Autodesk Inventor part; units mm, degrees
(part 3 of 3)
sketch "Sketch7" plane through (4.7625, 0, 0) normal (1, 0, 0) x (0, 0, -1)
  arc A0 (177.1237, 146.6426) -> (185.0928, 143.4752) centre (181.8846, 147.0122) ccw projected
  line L0 (177.1237, 146.6426) -> (173.518, 193.0979) projected
  arc A1 (175.8624, 197.5861) -> (173.518, 193.0979) centre (178.2789, 193.4674) ccw projected
  arc A2 (175.8624, 197.5861) -> (177.263, 198.4856) centre (165.4189, 215.3861) ccw projected
  arc A3 (182.3196, 198.751) -> (177.263, 198.4856) centre (180.0035, 194.5751) ccw projected
  line L1 (182.3196, 198.751) -> (208.3567, 184.3098) projected
  arc A4 (210.3177, 182.2574) -> (208.3567, 184.3098) centre (206.0406, 180.1339) ccw projected
  arc A5 (210.3177, 182.2574) -> (211.6131, 180.3381) centre (218.1439, 186.1428) ccw projected
  arc A6 (212.7982, 177.6127) -> (211.6131, 180.3381) centre (208.044, 177.1657) ccw projected
  arc A7 (212.7982, 177.6127) -> (213.775, 174.2825) centre (221.8723, 178.4659) ccw projected
  arc A8 (212.7408, 168.5537) -> (213.775, 174.2825) centre (209.5326, 172.0906) ccw projected
  line L2 (212.7408, 168.5537) -> (185.0928, 143.4752) projected
  line L3 (297.693, 129.8322) -> (298.103, 129.6534) projected
  arc A9 (300.9106, 126.0225) -> (298.103, 129.6534) centre (296.1941, 125.2763) ccw projected
  arc A10 (300.9106, 126.0225) -> (303.4157, 119.6426) centre (316.6157, 128.5073) ccw projected
  arc A11 (303.9033, 115.2529) -> (303.4157, 119.6426) centre (299.4515, 116.9804) ccw projected
  arc A12 (301.9596, 113.1838) -> (303.9033, 115.2529) centre (299.6083, 117.34) ccw projected
  arc A13 (301.9596, 113.1838) -> (301.3812, 112.8276) centre (306.462, 105.2251) ccw projected
  arc A14 (298.4626, 112.03) -> (301.3812, 112.8276) centre (298.7279, 116.7978) ccw projected
  line L4 (298.4626, 112.03) -> (288.0097, 112.6116) projected
  arc A15 (284.8365, 120.693) -> (288.0097, 112.6116) centre (288.275, 117.3794) ccw projected
  line L5 (284.8365, 120.693) -> (292.1012, 128.2313) projected
  arc A16 (294.7827, 129.6326) -> (292.1012, 128.2313) centre (295.5396, 124.9178) ccw projected
  arc A17 (294.7827, 129.6326) -> (296.0335, 129.9248) centre (293.3334, 138.661) ccw projected
  arc A18 (297.693, 129.8322) -> (296.0335, 129.9248) centre (296.7386, 127.6436) ccw projected
  arc A19 (103.3374, 74.4504) -> (106.8132, 70.7682) centre (108.0195, 75.3885) ccw projected
  line L6 (103.3374, 74.4504) -> (95.1658, 115.2322) projected
  arc A20 (96.9547, 119.9692) -> (95.1658, 115.2322) centre (99.848, 116.1703) ccw projected
  arc A21 (96.9547, 119.9692) -> (101.5055, 124.7667) centre (84.4507, 136.3874) ccw projected
  arc A22 (106.1416, 126.803) -> (101.5055, 124.7667) centre (105.4517, 122.0779) ccw projected
  line L7 (106.1416, 126.803) -> (150.0332, 120.3943) projected
  arc A23 (152.7613, 112.3346) -> (150.0332, 120.3943) centre (149.3433, 115.6692) ccw projected
  line L8 (152.7613, 112.3346) -> (113.01, 71.5887) projected
  arc A24 (108.0902, 70.3904) -> (113.01, 71.5887) centre (109.5919, 74.9233) ccw projected
  arc A25 (108.0902, 70.3904) -> (106.8132, 70.7682) centre (101.6, 50.8) ccw projected
  arc A26 (79.5512, 19.1063) -> (80.7269, 11.5557) centre (82.9692, 15.7717) ccw projected
  line L9 (79.5512, 19.1063) -> (90.19, 30.0113) projected
  arc A27 (95.1098, 31.2096) -> (90.19, 30.0113) centre (93.6081, 26.6767) ccw projected
  arc A28 (95.1098, 31.2096) -> (99.5296, 30.2666) centre (101.6, 50.8) ccw projected
  arc A29 (103.5319, 27.1647) -> (99.5296, 30.2666) centre (99.0506, 25.5155) ccw projected
  line L10 (103.5319, 27.1647) -> (107.8479, 15.4373) projected
  arc A30 (107.879, 12.226) -> (107.8479, 15.4373) centre (103.3665, 13.7881) ccw projected
  arc A31 (107.879, 12.226) -> (107.4494, 10.4582) centre (116.952, 9.0853) ccw projected
  arc A32 (102.8585, 6.3678) -> (107.4494, 10.4582) centre (102.7233, 11.1411) ccw projected
  arc A33 (80.7269, 11.5557) -> (102.8585, 6.3678) centre (101.6, 50.8) ccw projected
  arc A34 (119.7664, 19.8236) -> (121.8244, 17.3583) centre (124.2477, 21.4729) ccw projected
  line L11 (119.7664, 19.8236) -> (115.4504, 31.551) projected
  arc A35 (116.4871, 36.5074) -> (115.4504, 31.551) centre (119.9318, 33.2003) ccw projected
  arc A36 (116.4871, 36.5074) -> (120.5052, 42.5235) centre (101.6, 50.8) ccw projected
  arc A37 (124.6863, 45.3797) -> (120.5052, 42.5235) centre (124.8796, 40.6084) ccw projected
  line L12 (124.6863, 45.3797) -> (179.7658, 47.6103) projected
  arc A38 (181.9351, 38.4919) -> (179.7658, 47.6103) centre (179.959, 42.839) ccw projected
  line L13 (181.9351, 38.4919) -> (129.3853, 14.6036) projected
  arc A39 (123.9358, 15.6738) -> (129.3853, 14.6036) centre (127.4092, 18.9507) ccw projected
  arc A40 (123.9358, 15.6738) -> (121.8244, 17.3583) centre (116.952, 9.0853) ccw projected
  arc A41 (269.7893, 127.2498) -> (264.2711, 128.2398) centre (263.4194, 107.6199) ccw projected
  arc A42 (260.0922, 131.0994) -> (264.2711, 128.2398) centre (264.4682, 133.011) ccw projected
  line L14 (260.0922, 131.0994) -> (256.6371, 139.0089) projected
  arc A43 (262.9615, 145.28) -> (256.6371, 139.0089) centre (261.013, 140.9204) ccw projected
  line L15 (262.9615, 145.28) -> (276.2747, 139.3298) projected
  arc A44 (277.7647, 131.6567) -> (276.2747, 139.3298) centre (274.3263, 134.9702) ccw projected
  line L16 (277.7647, 131.6567) -> (274.7017, 128.4782) projected
  arc A45 (269.7893, 127.2498) -> (274.7017, 128.4782) centre (271.2632, 131.7918) ccw projected
  arc A46 (114.238, 194.0376) -> (111.6305, 192.1628) centre (115.5595, 189.4489) ccw projected
  line L17 (114.238, 194.0376) -> (145.2207, 202.9608) projected
  arc A47 (150.0893, 201.5691) -> (145.2207, 202.9608) centre (146.5423, 198.3721) ccw projected
  arc A48 (150.0893, 201.5691) -> (157.8472, 196.1878) centre (165.4189, 215.3861) ccw projected
  arc A49 (160.8561, 192.1151) -> (157.8472, 196.1878) centre (156.0952, 191.7456) ccw projected
  line L18 (160.8561, 192.1151) -> (165.1407, 136.9136) projected
  arc A50 (159.6899, 131.819) -> (165.1407, 136.9136) centre (160.3798, 136.5441) ccw projected
  line L19 (159.6899, 131.819) -> (107.9765, 139.3697) projected
  arc A51 (104.1161, 142.6465) -> (107.9765, 139.3697) centre (108.6664, 144.0948) ccw projected
  arc A52 (104.1161, 142.6465) -> (98.6409, 151.3722) centre (84.4507, 136.3874) ccw projected
  arc A53 (97.3696, 156.2736) -> (98.6409, 151.3722) centre (101.9243, 154.8395) ccw projected
  line L20 (97.3696, 156.2736) -> (107.0529, 187.0272) projected
  arc A54 (108.9913, 189.5877) -> (107.0529, 187.0272) centre (111.6076, 185.5931) ccw projected
  arc A55 (108.9913, 189.5877) -> (111.6305, 192.1628) centre (103.7307, 197.6195) ccw projected
  arc A56 (247.7126, 121.0065) -> (248.4542, 126.0155) centre (244.0783, 124.104) ccw projected
  arc A57 (247.7126, 121.0065) -> (246.7001, 119.7182) centre (263.4194, 107.6199) ccw projected
  arc A58 (242.0082, 117.8138) -> (246.7001, 119.7182) centre (242.8314, 122.5175) ccw projected
  line L21 (242.0082, 117.8138) -> (196.0441, 125.8585) projected
  arc A59 (193.6591, 134.0992) -> (196.0441, 125.8585) centre (196.8673, 130.5622) ccw projected
  line L22 (193.6591, 134.0992) -> (221.2962, 159.1677) projected
  arc A60 (227.1405, 159.6124) -> (221.2962, 159.1677) centre (224.5044, 155.6308) ccw projected
  arc A61 (227.1405, 159.6124) -> (230.3016, 158.322) centre (231.9501, 166.8768) ccw projected
  arc A62 (232.9035, 156.8757) -> (230.3016, 158.322) centre (229.3981, 153.633) ccw projected
  arc A63 (232.9035, 156.8757) -> (234.7042, 155.389) centre (239.3128, 162.8049) ccw projected
  arc A64 (236.5596, 153.2447) -> (234.7042, 155.389) centre (232.1837, 151.3332) ccw projected
  line L23 (236.5596, 153.2447) -> (248.4542, 126.0155) projected
  arc A65 (246.6512, 77.8946) -> (252.2773, 70.4684) centre (250.3012, 74.8155) ccw projected
  line L24 (246.6512, 77.8946) -> (253.5407, 86.0614) projected
  arc A66 (258.3611, 87.6119) -> (253.5407, 86.0614) centre (257.1906, 82.9824) ccw projected
  arc A67 (258.3611, 87.6119) -> (281.4437, 97.5684) centre (263.4194, 107.6199) ccw projected
  arc A68 (285.8795, 100.0105) -> (281.4437, 97.5684) centre (285.6142, 95.2426) ccw projected
  line L25 (285.8795, 100.0105) -> (292.479, 99.6433) projected
  arc A69 (294.3831, 90.6215) -> (292.479, 99.6433) centre (292.2137, 94.8754) ccw projected
  line L26 (294.3831, 90.6215) -> (276.6898, 81.5983) projected
  arc A70 (275.5075, 81.0285) -> (276.6898, 81.5983) centre (263.4194, 107.6199) ccw projected
  line L27 (275.5075, 81.0285) -> (252.2773, 70.4684) projected
  arc A71 (71.645, 102.7043) -> (71.6097, 103.9717) centre (62.0508, 103.0707) ccw projected
  arc A72 (72.401, 107.0842) -> (71.6097, 103.9717) centre (76.3638, 104.4199) ccw projected
  line L28 (72.401, 107.0842) -> (74.8246, 110.689) projected
  arc A73 (83.4696, 108.9629) -> (74.8246, 110.689) centre (78.7874, 108.0247) ccw projected
  line L29 (83.4696, 108.9629) -> (85.8233, 97.2162) projected
  arc A74 (77.3331, 93.3968) -> (85.8233, 97.2162) centre (81.1411, 96.278) ccw projected
  line L30 (77.3331, 93.3968) -> (72.6087, 99.6409) projected
  arc A75 (71.645, 102.7043) -> (72.6087, 99.6409) centre (76.4168, 102.5221) ccw projected
  arc A76 (62.8834, 28.9637) -> (70.4607, 27.9749) centre (67.0427, 31.3095) ccw projected
  arc A77 (57.3611, 55.1273) -> (62.8834, 28.9637) centre (101.6, 50.8) ccw projected
  line L31 (57.3611, 55.1273) -> (59.9499, 81.5928) projected
  arc A78 (68.5105, 84.0091) -> (59.9499, 81.5928) centre (64.7024, 81.1279) ccw projected
  line L32 (68.5105, 84.0091) -> (82.7502, 65.189) projected
  arc A79 (83.1997, 60.1454) -> (82.7502, 65.189) centre (78.9422, 62.3077) ccw projected
  arc A80 (83.1997, 60.1454) -> (82.1759, 43.8278) centre (101.6, 50.8) ccw projected
  arc A81 (81.0995, 38.8799) -> (82.1759, 43.8278) centre (77.6815, 42.2145) ccw projected
  line L33 (81.0995, 38.8799) -> (70.4607, 27.9749) projected
  arc A82 (125.6733, 66.3823) -> (129.2845, 58.2764) centre (129.0913, 63.0477) ccw projected
  line L34 (125.6733, 66.3823) -> (167.6605, 109.42) projected
  arc A83 (175.0067, 108.8006) -> (167.6605, 109.42) centre (171.0785, 106.0854) ccw projected
  line L35 (175.0067, 108.8006) -> (202.8011, 68.5888) projected
  arc A84 (199.0662, 61.1024) -> (202.8011, 68.5888) centre (198.8729, 65.8737) ccw projected
  line L36 (199.0662, 61.1024) -> (129.2845, 58.2764) projected
  arc A85 (197.6387, 112.6864) -> (192.8872, 105.2675) centre (196.8154, 107.9827) ccw projected
  line L37 (197.6387, 112.6864) -> (239.8187, 105.304) projected
  arc A86 (243.5849, 101.9193) -> (239.8187, 105.304) centre (238.9955, 100.6003) ccw projected
  arc A87 (243.5849, 101.9193) -> (244.5496, 99.2631) centre (263.4194, 107.6199) ccw projected
  arc A88 (243.8334, 94.2504) -> (244.5496, 99.2631) centre (240.1835, 97.3294) ccw projected
  line L38 (243.8334, 94.2504) -> (224.0438, 70.7914) projected
  arc A89 (216.4656, 71.1553) -> (224.0438, 70.7914) centre (220.3938, 73.8705) ccw projected
  line L39 (216.4656, 71.1553) -> (192.8872, 105.2675) projected
  arc A90 (117.1001, 216.8987) -> (122.3457, 209.5888) centre (121.0241, 214.1775) ccw projected
  line L40 (117.1001, 216.8987) -> (136.9001, 245.4509) projected
  arc A91 (139.8047, 246.284) -> (136.9001, 245.4509) centre (138.8621, 244.0903) ccw projected
  arc A92 (139.8047, 246.284) -> (140.0117, 246.1979) centre (143.5951, 255.1053) ccw projected
  arc A93 (142.4146, 244.0672) -> (140.0117, 246.1979) centre (138.2295, 241.7677) ccw projected
  line L41 (142.4146, 244.0672) -> (148.8512, 232.3527) projected
  arc A94 (148.5657, 227.2972) -> (148.8512, 232.3527) centre (144.6661, 230.0532) ccw projected
  arc A95 (148.5657, 227.2972) -> (145.0885, 218.9327) centre (165.4189, 215.3861) ccw projected
  arc A96 (141.7059, 215.1647) -> (145.0885, 218.9327) centre (140.3843, 219.7534) ccw projected
  line L42 (141.7059, 215.1647) -> (122.3457, 209.5888) projected
  arc A97 (170.8837, 294.4565) -> (172.0866, 287.8113) centre (174.8077, 291.7353) ccw projected
  line L43 (170.8837, 294.4565) -> (172.7922, 297.2086) projected
  arc A98 (174.2704, 299.1942) -> (172.7922, 297.2086) centre (203.0571, 276.2209) ccw projected
  line L44 (174.2704, 299.1942) -> (186.7738, 314.8615) projected
  arc A99 (195.2416, 312.4978) -> (186.7738, 314.8615) centre (190.5061, 311.8829) ccw projected
  line L45 (195.2416, 312.4978) -> (195.6829, 309.0987) projected
  arc A100 (195.1019, 306.1294) -> (195.6829, 309.0987) centre (190.9475, 308.4838) ccw projected
  arc A101 (195.1019, 306.1294) -> (196.1286, 295.6536) centre (203.0571, 301.6209) ccw projected
  arc A102 (196.7071, 294.0954) -> (196.1286, 295.6536) centre (194.3195, 294.0954) ccw projected
  line L46 (196.7071, 294.0954) -> (196.7071, 292.4021) projected
  arc A103 (195.454, 290.3012) -> (196.7071, 292.4021) centre (194.3195, 292.4021) ccw projected
  arc A104 (195.454, 290.3012) -> (188.9768, 283.824) centre (203.0571, 276.2209) ccw projected
  arc A105 (186.8759, 282.5709) -> (188.9768, 283.824) centre (186.8759, 284.9585) ccw projected
  line L47 (186.8759, 282.5709) -> (186.0222, 282.5709) projected
  arc A106 (183.1524, 283.5294) -> (186.0222, 282.5709) centre (186.0222, 287.3461) ccw projected
  arc A107 (183.1524, 283.5294) -> (177.3062, 285.3581) centre (177.6571, 276.2209) ccw projected
  arc A108 (174.4018, 286.2058) -> (177.3062, 285.3581) centre (177.1229, 290.1298) ccw projected
  line L48 (174.4018, 286.2058) -> (172.0866, 287.8113) projected
  arc A109 (298.3468, 346.8044) -> (302.3019, 353.3428) centre (297.8735, 351.556) ccw projected
  line L49 (298.3468, 346.8044) -> (283.1869, 345.2944) projected
  arc A110 (278.6486, 347.5403) -> (283.1869, 345.2944) centre (282.7136, 350.046) ccw projected
  arc A111 (278.6486, 347.5403) -> (268.2318, 356.07) centre (261.0807, 336.7111) ccw projected
  arc A112 (265.1348, 360.076) -> (268.2318, 356.07) centre (269.8865, 360.5493) ccw projected
  line L50 (265.1348, 360.076) -> (263.6248, 375.236) projected
  arc A113 (269.2547, 380.403) -> (263.6248, 375.236) centre (268.3765, 375.7093) ccw projected
  arc A114 (302.3019, 353.3428) -> (269.2547, 380.403) centre (261.0807, 336.7111) ccw projected
  arc A115 (379.8681, 143.7131) -> (386.4173, 137.5565) centre (384.2479, 141.8105) ccw projected
  line L51 (379.8681, 143.7131) -> (390.24, 167.5887) projected
  arc A116 (394.413, 170.4568) -> (390.24, 167.5887) centre (394.6197, 165.686) ccw projected
  arc A117 (394.413, 170.4568) -> (413.0231, 184.3286) centre (393.5194, 191.0749) ccw projected
  arc A118 (416.9638, 187.5084) -> (413.0231, 184.3286) centre (417.536, 182.7676) ccw projected
  line L52 (416.9638, 187.5084) -> (432.089, 189.3339) projected
  arc A119 (437.3722, 183.813) -> (432.089, 189.3339) centre (432.6612, 184.5931) ccw projected
  arc A120 (413.7134, 151.4769) -> (437.3722, 183.813) centre (393.5194, 191.0749) ccw projected
  line L53 (413.7134, 151.4769) -> (386.4173, 137.5565) projected
  arc A121 (430.5672, 201.9424) -> (434.3852, 208.5618) centre (429.995, 206.6832) ccw projected
  line L54 (430.5672, 201.9424) -> (415.442, 200.1169) projected
  arc A122 (410.858, 202.2678) -> (415.442, 200.1169) centre (414.8698, 204.8577) ccw projected
  arc A123 (410.858, 202.2678) -> (400.2657, 210.5786) centre (393.5194, 191.0749) ccw projected
  arc A124 (397.0859, 214.5193) -> (400.2657, 210.5786) centre (401.8267, 215.0914) ccw projected
  line L55 (397.0859, 214.5193) -> (395.2604, 229.6445) projected
  arc A125 (400.7814, 234.9277) -> (395.2604, 229.6445) centre (400.0012, 230.2167) ccw projected
  arc A126 (434.3852, 208.5618) -> (400.7814, 234.9277) centre (393.5194, 191.0749) ccw projected
  arc A127 (250.9874, 373.9773) -> (244.449, 377.9323) centre (246.2357, 373.504) ccw projected
  line L56 (250.9874, 373.9773) -> (252.4974, 358.8173) projected
  arc A128 (250.2514, 354.2791) -> (252.4974, 358.8173) centre (247.7457, 358.344) ccw projected
  arc A129 (250.2514, 354.2791) -> (241.7218, 343.8623) centre (261.0807, 336.7111) ccw projected
  arc A130 (237.7157, 340.7653) -> (241.7218, 343.8623) centre (237.2424, 345.5169) ccw projected
  line L57 (237.7157, 340.7653) -> (216.1032, 338.6126) projected
  arc A131 (211.8976, 346.3429) -> (216.1032, 338.6126) centre (215.6299, 343.3643) ccw projected
  line L58 (211.8976, 346.3429) -> (226.3381, 364.4375) projected
  arc A132 (244.449, 377.9323) -> (226.3381, 364.4375) centre (261.0807, 336.7111) ccw projected
  arc A133 (198.999, 204.1865) -> (205.9543, 209.4304) centre (201.2979, 208.3719) ccw projected
  line L59 (198.999, 204.1865) -> (188.5021, 209.9521) projected
  arc A134 (186.0315, 214.3721) -> (188.5021, 209.9521) centre (190.801, 214.1375) ccw projected
  arc A135 (186.0315, 214.3721) -> (185.1217, 221.5267) centre (165.4189, 215.3861) ccw projected
  arc A136 (186.4073, 226.4244) -> (185.1217, 221.5267) centre (189.6806, 222.9476) ccw projected
  line L60 (186.4073, 226.4244) -> (193.2473, 232.864) projected
  arc A137 (201.177, 230.4457) -> (193.2473, 232.864) centre (196.5206, 229.3871) ccw projected
  line L61 (201.177, 230.4457) -> (205.9543, 209.4304) projected
  arc A138 (211.3352, 325.3748) -> (207.073, 320.0083) centre (211.8085, 320.6231) ccw projected
  line L62 (211.3352, 325.3748) -> (238.9744, 328.1278) projected
  arc A139 (243.5127, 325.8818) -> (238.9744, 328.1278) centre (239.4477, 323.3761) ccw projected
  arc A140 (243.5127, 325.8818) -> (244.321, 324.6686) centre (261.0807, 336.7111) ccw projected
  arc A141 (244.646, 319.6154) -> (244.321, 324.6686) centre (240.4431, 321.8822) ccw projected
  line L63 (244.646, 319.6154) -> (226.8389, 286.5977) projected
  arc A142 (224.633, 284.5268) -> (226.8389, 286.5977) centre (222.636, 288.8644) ccw projected
  arc A143 (224.633, 284.5268) -> (222.4898, 283.1494) centre (228.4571, 276.2209) ccw projected
  arc A144 (220.9317, 282.5709) -> (222.4898, 283.1494) centre (220.9317, 284.9585) ccw projected
  line L64 (220.9317, 282.5709) -> (219.2384, 282.5709) projected
  arc A145 (217.1375, 283.824) -> (219.2384, 282.5709) centre (219.2384, 284.9585) ccw projected
  arc A146 (217.1375, 283.824) -> (210.6603, 290.3012) centre (203.0571, 276.2209) ccw projected
  arc A147 (209.4071, 292.4021) -> (210.6603, 290.3012) centre (211.7947, 292.4021) ccw projected
  line L65 (209.4071, 292.4021) -> (209.4071, 294.0954) projected
  arc A148 (209.9856, 295.6536) -> (209.4071, 294.0954) centre (211.7947, 294.0954) ccw projected
  arc A149 (209.9856, 295.6536) -> (209.5973, 308.0115) centre (203.0571, 301.6209) ccw projected
  arc A150 (208.2772, 310.7339) -> (209.5973, 308.0115) centre (213.0127, 311.3488) ccw projected
  line L66 (208.2772, 310.7339) -> (207.073, 320.0083) projected
  arc A151 (219.2384, 269.8709) -> (217.1375, 268.6177) centre (219.2384, 267.4833) ccw projected
  line L67 (219.2384, 269.8709) -> (220.9317, 269.8709) projected
  arc A152 (222.4898, 269.2924) -> (220.9317, 269.8709) centre (220.9317, 267.4833) ccw projected
  arc A153 (222.4898, 269.2924) -> (232.2342, 267.8934) centre (228.4571, 276.2209) ccw projected
  arc A154 (235.2436, 268.2059) -> (232.2342, 267.8934) centre (234.2067, 263.5446) ccw projected
  line L68 (235.2436, 268.2059) -> (318.0387, 249.787) projected
  arc A155 (321.7764, 245.0563) -> (318.0387, 249.787) centre (317.0017, 245.1258) ccw projected
  line L69 (321.7764, 245.0563) -> (320.5418, 160.2462) projected
  arc A156 (319.5416, 157.3907) -> (320.5418, 160.2462) centre (315.7671, 160.3157) ccw projected
  arc A157 (319.5416, 157.3907) -> (317.8734, 149.6741) centre (326.7693, 151.7896) ccw projected
  arc A158 (317.6048, 146.6604) -> (317.8734, 149.6741) centre (313.2278, 148.5693) ccw projected
  line L70 (317.6048, 146.6604) -> (317.2174, 145.7719) projected
  arc A159 (315.236, 144.3478) -> (317.2174, 145.7719) centre (315.0288, 146.7264) ccw projected
  arc A160 (315.236, 144.3478) -> (306.8489, 141.0546) centre (316.6157, 128.5073) ccw projected
  arc A161 (304.4279, 140.7502) -> (306.8489, 141.0546) centre (305.3824, 142.9387) ccw projected
  line L71 (304.4279, 140.7502) -> (302.7698, 141.4733) projected
  arc A162 (301.5729, 142.6264) -> (302.7698, 141.4733) centre (303.7243, 143.6618) ccw projected
  arc A163 (301.5729, 142.6264) -> (291.2986, 147.5757) centre (293.3334, 138.661) ccw projected
  arc A164 (288.2875, 147.8716) -> (291.2986, 147.5757) centre (290.2359, 152.2312) ccw projected
  line L72 (288.2875, 147.8716) -> (248.8959, 165.4772) projected
  arc A165 (246.7674, 167.3507) -> (248.8959, 165.4772) centre (250.8444, 169.8368) ccw projected
  arc A166 (246.7674, 167.3507) -> (245.8371, 168.6073) centre (239.3128, 162.8049) ccw projected
  arc A167 (244.6507, 171.3375) -> (245.8371, 168.6073) centre (249.4053, 171.7808) ccw projected
  arc A168 (244.6507, 171.3375) -> (242.4292, 176.382) centre (235.9761, 170.5287) ccw projected
  line L73 (242.4292, 176.382) -> (231.9513, 187.9335) projected
  arc A169 (231.9513, 187.9335) -> (227.1533, 190.6337) centre (225.4982, 182.0802) ccw projected
  arc A170 (224.5561, 192.0782) -> (227.1533, 190.6337) centre (228.0605, 195.3219) ccw projected
  arc A171 (224.5561, 192.0782) -> (223.7494, 192.8453) centre (218.1439, 186.1428) ccw projected
  arc A172 (222.1565, 195.4498) -> (223.7494, 192.8453) centre (226.8129, 196.5083) ccw projected
  line L74 (222.1565, 195.4498) -> (211.1035, 244.0716) projected
  arc A173 (211.402, 247.0824) -> (211.1035, 244.0716) centre (215.7599, 245.1301) ccw projected
  arc A174 (211.402, 247.0824) -> (209.9856, 256.7882) centre (203.0571, 250.8209) ccw projected
  arc A175 (209.4071, 258.3463) -> (209.9856, 256.7882) centre (211.7947, 258.3463) ccw projected
  line L75 (209.4071, 258.3463) -> (209.4071, 260.0397) projected
  arc A176 (210.6603, 262.1405) -> (209.4071, 260.0397) centre (211.7947, 260.0397) ccw projected
  arc A177 (210.6603, 262.1405) -> (217.1375, 268.6177) centre (203.0571, 276.2209) ccw projected
  arc A178 (337.1993, 150.5599) -> (335.2123, 148.2783) centre (339.6214, 146.4446) ccw projected
  line L76 (337.1993, 150.5599) -> (367.2672, 168.2562) projected
  arc A179 (374.069, 162.2382) -> (367.2672, 168.2562) centre (369.6893, 164.1408) ccw projected
  line L77 (374.069, 162.2382) -> (363.4789, 137.8602) projected
  arc A180 (361.2833, 135.5164) -> (363.4789, 137.8602) centre (359.0991, 139.7628) ccw projected
  arc A181 (361.2833, 135.5164) -> (357.5507, 132.0949) centre (365.675, 126.9785) ccw projected
  arc A182 (355.0252, 130.1112) -> (357.5507, 132.0949) centre (353.51, 134.6396) ccw projected
  line L78 (355.0252, 130.1112) -> (345.8158, 127.0298) projected
  arc A183 (342.7902, 127.0282) -> (345.8158, 127.0298) centre (344.3006, 131.5582) ccw projected
  arc A184 (342.7902, 127.0282) -> (337.1978, 127.0899) centre (339.8979, 118.3537) ccw projected
  arc A185 (335.5383, 127.1825) -> (337.1978, 127.0899) centre (336.4928, 129.3711) ccw projected
  line L79 (335.5383, 127.1825) -> (335.1284, 127.3613) projected
  arc A186 (332.3207, 130.9922) -> (335.1284, 127.3613) centre (337.0372, 131.7384) ccw projected
  arc A187 (332.3207, 130.9922) -> (329.1629, 138.2741) centre (316.6157, 128.5073) ccw projected
  arc A188 (328.8585, 140.6951) -> (329.1629, 138.2741) centre (331.047, 139.7406) ccw projected
  line L80 (328.8585, 140.6951) -> (329.246, 141.5836) projected
  arc A189 (331.2718, 143.8309) -> (329.246, 141.5836) centre (333.623, 139.6747) ccw projected
  arc A190 (331.2718, 143.8309) -> (335.2123, 148.2783) centre (326.7693, 151.7896) ccw projected
  arc A191 (382.3265, 208.4134) -> (384.4774, 212.9975) centre (379.7366, 212.4253) ccw projected
  arc A192 (382.3265, 208.4134) -> (372.946, 189.4499) centre (393.5194, 191.0749) ccw projected
  arc A193 (370.6077, 184.9585) -> (372.946, 189.4499) centre (368.1856, 189.0739) ccw projected
  line L81 (370.6077, 184.9585) -> (340.6035, 167.2997) projected
  arc A194 (333.4067, 171.4846) -> (340.6035, 167.2997) centre (338.1814, 171.4151) ccw projected
  line L82 (333.4067, 171.4846) -> (334.4104, 240.4277) projected
  arc A195 (341.5331, 244.5162) -> (334.4104, 240.4277) centre (339.1851, 240.3582) ccw projected
  arc A196 (341.5331, 244.5162) -> (377.7123, 234.6667) centre (379.0508, 310.9542) ccw projected
  arc A197 (382.3693, 230.4644) -> (377.7123, 234.6667) centre (377.6285, 229.8922) ccw projected
  line L83 (382.3693, 230.4644) -> (384.4774, 212.9975) projected
  arc A198 (241.0284, 286.1531) -> (244.1944, 279.2252) centre (245.2313, 283.8864) ccw projected
  line L84 (241.0284, 286.1531) -> (255.824, 313.5869) projected
  arc A199 (260.2249, 316.0913) -> (255.824, 313.5869) centre (260.0269, 311.3202) ccw projected
  arc A200 (260.2249, 316.0913) -> (280.4395, 329.5599) centre (261.0807, 336.7111) ccw projected
  arc A201 (284.4456, 332.6569) -> (280.4395, 329.5599) centre (284.9189, 327.9052) ccw projected
  line L85 (284.4456, 332.6569) -> (299.6056, 334.1669) projected
  arc A202 (304.7726, 328.5371) -> (299.6056, 334.1669) centre (300.0789, 329.4152) ccw projected
  arc A203 (304.5076, 327.2295) -> (304.7726, 328.5371) centre (261.0807, 336.7111) ccw projected
  arc A204 (304.5076, 327.2295) -> (313.4045, 272.0681) centre (379.0508, 310.9542) ccw projected
  arc A205 (308.259, 264.9731) -> (313.4045, 272.0681) centre (309.296, 269.6344) ccw projected
  line L86 (308.259, 264.9731) -> (244.1944, 279.2252) projected
  arc A206 (185.1826, 269.8709) -> (183.6244, 269.2924) centre (185.1826, 267.4833) ccw projected
  line L87 (185.1826, 269.8709) -> (185.5094, 269.8709) projected
  arc A207 (189.5424, 267.6526) -> (185.5094, 269.8709) centre (185.5094, 265.0957) ccw projected
  arc A208 (189.5424, 267.6526) -> (195.454, 262.1405) centre (203.0571, 276.2209) ccw projected
  arc A209 (196.7071, 260.0397) -> (195.454, 262.1405) centre (194.3195, 260.0397) ccw projected
  line L88 (196.7071, 260.0397) -> (196.7071, 259.1859) projected
  arc A210 (195.7486, 256.3162) -> (196.7071, 259.1859) centre (191.9319, 259.1859) ccw projected
  arc A211 (195.7486, 256.3162) -> (194.0462, 252.3753) centre (203.0571, 250.8209) ccw projected
  arc A212 (192.6138, 249.7103) -> (194.0462, 252.3753) centre (189.3405, 253.1871) ccw projected
  line L89 (192.6138, 249.7103) -> (177.7018, 235.6713) projected
  arc A213 (172.7356, 234.683) -> (177.7018, 235.6713) centre (174.4285, 239.1481) ccw projected
  arc A214 (172.7356, 234.683) -> (164.402, 235.9985) centre (165.4189, 215.3861) ccw projected
  arc A215 (159.9817, 238.4684) -> (164.402, 235.9985) centre (164.1668, 240.7679) ccw projected
  line L90 (159.9817, 238.4684) -> (154.2435, 248.9118) projected
  arc A216 (155.9126, 255.2699) -> (154.2435, 248.9118) centre (158.4286, 251.2113) ccw projected
  line L91 (155.9126, 255.2699) -> (173.8931, 266.4164) projected
  arc A217 (176.8373, 267.1137) -> (173.8931, 266.4164) centre (176.4091, 262.3577) ccw projected
  arc A218 (176.8373, 267.1137) -> (183.6244, 269.2924) centre (177.6571, 276.2209) ccw projected
  circle A219 centre (62.0508, 103.0707) radius 3.2512 projected
  circle A220 centre (365.675, 126.9785) radius 3.2512 projected
  circle A221 centre (116.952, 9.0853) radius 3.2512 projected
  circle A222 centre (143.5951, 255.1053) radius 3.2512 projected
  circle A223 centre (199.3, 330.5575) radius 3.2512 projected
  circle A224 centre (219.5153, 55.5753) radius 3.2512 projected
  line L92 (167.5741, 300.8271) -> (63.5783, 150.8617) projected
  arc A225 (63.5783, 150.8617) -> (59.1713, 138.8602) centre (84.4507, 136.3874) ccw projected
  line L93 (59.1713, 138.8602) -> (51.0413, 55.7455) projected
  arc A226 (51.0413, 55.7455) -> (122.6227, 4.5541) centre (101.6, 50.8) ccw projected
  line L94 (122.6227, 4.5541) -> (278.1353, 75.2478) projected
  arc A227 (278.1353, 75.2478) -> (279.5746, 75.9415) centre (263.4194, 107.6199) ccw projected
  line L95 (279.5746, 75.9415) -> (416.5983, 145.82) projected
  arc A228 (416.5983, 145.82) -> (387.4324, 241.5089) centre (393.5194, 191.0749) ccw projected
  arc A229 (310.7115, 325.875) -> (387.4324, 241.5089) centre (379.0508, 310.9542) ccw projected
  arc A230 (310.7115, 325.875) -> (221.3748, 368.3984) centre (261.0807, 336.7111) ccw projected
  line L96 (221.3748, 368.3984) -> (169.3072, 303.1551) projected
  arc A231 (169.3072, 303.1551) -> (167.5741, 300.8271) centre (203.0571, 276.2209) ccw projected
  circle A232 centre (326.7693, 151.7896) radius 2.794 projected
  circle A233 centre (172.549, 123.5241) radius 3.2512 projected
  circle A234 centre (203.0571, 276.2209) radius 9.652 projected
  circle A235 centre (228.4571, 276.2209) radius 2.794 projected
  circle A236 centre (203.0571, 250.8209) radius 2.794 projected
  circle A237 centre (177.6571, 276.2209) radius 2.794 projected
  circle A238 centre (84.4507, 136.3874) radius 14.2875 projected
  circle A239 centre (263.4194, 107.6199) radius 14.2875 projected
  circle A240 centre (316.6157, 128.5073) radius 9.5504 projected
  circle A241 centre (239.3128, 162.8049) radius 2.3812 projected
  circle A242 centre (218.1439, 186.1428) radius 2.3876 projected
  arc A243 (219.8851, 180.1779) -> (219.7225, 176.8412) centre (221.4722, 178.4283) ccw projected
  line L97 (219.8851, 180.1779) -> (223.9112, 183.8298) projected
  arc A244 (227.2479, 183.6672) -> (223.9112, 183.8298) centre (225.4982, 182.0802) ccw projected
  line L98 (227.2479, 183.6672) -> (237.7258, 172.1157) projected
  arc A245 (237.5632, 168.779) -> (237.7258, 172.1157) centre (235.9761, 170.5287) ccw projected
  line L99 (237.5632, 168.779) -> (233.5371, 165.1271) projected
  arc A246 (230.2004, 165.2897) -> (233.5371, 165.1271) centre (231.9501, 166.8768) ccw projected
  line L100 (230.2004, 165.2897) -> (219.7225, 176.8412) projected
  circle A247 centre (339.8979, 118.3537) radius 2.794 projected
  circle A248 centre (306.462, 105.2251) radius 2.794 projected
  circle A249 centre (293.3334, 138.661) radius 2.794 projected
  circle A250 centre (103.7307, 197.6195) radius 3.2512 projected
  circle A251 centre (203.0571, 301.6209) radius 2.794 projected
  circle A252 centre (101.6, 50.8) radius 14.2875 projected
  circle A253 centre (165.4189, 215.3861) radius 14.2875 projected
  circle A254 centre (393.5194, 191.0749) radius 14.2875 projected
  circle A255 centre (261.0807, 336.7111) radius 14.2875 projected
  point P0 (0, 0)
body "Solid3"
